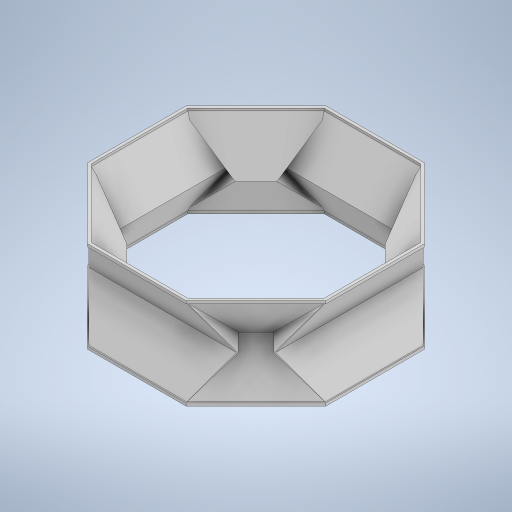
# Autodesk Inventor part: 팔각형 OV-PAM 층 한개
Saved by Autodesk Inventor 2024 (Build 280153000, 153)
## iProperties
Created: 2023-06-16
Part Number: 팔각형 OV-PAM 층 한개
Material: 일반
Document SubType Name: Modeling
Designer: jsw
Density: 1 g/cm^3
Appearance: 기본값
Author: jsw
Autodesk Inventor part; units mm, degrees
ref_plane "YZ Plane" through (0, 0, 0) normal (1, 0, 0) x (0, 1, 0)
ref_plane "XZ Plane" through (0, 0, 0) normal (0, 1, 0) x (-1, 0, 0)
ref_plane "XY Plane" through (0, 0, 0) normal (0, 0, 1) x (1, 0, 0)
sketch "스케치1" plane through (0, 0, 0) normal (0, 1, 0) x (-1, 0, 0)
  line L0 (-32.5919, 13.5) -> (-13.5, 32.5919)
  line L1 (-13.5, 32.5919) -> (13.5, 32.5919)
  line L2 (13.5, 32.5919) -> (32.5919, 13.5)
  line L3 (32.5919, 13.5) -> (32.5919, -13.5)
  line L4 (32.5919, -13.5) -> (13.5, -32.5919)
  line L5 (13.5, -32.5919) -> (-13.5, -32.5919)
  line L6 (-13.5, -32.5919) -> (-32.5919, -13.5)
  line L7 (-32.5919, -13.5) -> (-32.5919, 13.5)
  line L8 (-13.7071, 33.0919) -> (13.7071, 33.0919)
  line L9 (13.7071, 33.0919) -> (33.0919, 13.7071)
  line L10 (33.0919, 13.7071) -> (33.0919, -13.7071)
  line L11 (33.0919, -13.7071) -> (13.7071, -33.0919)
  line L12 (13.7071, -33.0919) -> (-13.7071, -33.0919)
  line L13 (-13.7071, -33.0919) -> (-33.0919, -13.7071)
  line L14 (-33.0919, -13.7071) -> (-33.0919, 13.7071)
  line L15 (-33.0919, 13.7071) -> (-13.7071, 33.0919)
  point P0 (0, 0)
  point P1 (0, 0)
  point P2 (0, 0)
  dimension "d0" = 27
  dimension "d2" = 0.5
  constraints: 32 end point, 2 coincident, 2 horizontal, 34 other
  measures "d0" distance of L0.end L1.end
  measures "d2" distance between parallel lines of L10 L3
extrude "돌출2" add sketch "스케치1" along normal blind 12 contours L0 L1 L2 L3 L4 L5 L6 L7 | L8 L9 L10 L11 L12 L13 L14 L15
ref_plane "작업 평면2" through (33.0919, 0, 13.7071) normal (-0.8660254, -0.5, 0) x (0, 0, -1)
sketch "스케치3" plane through (33.0919, 0, 13.7071) normal (1, 0, 0) x (0, 0, -1)
  line L0 (0, 0) -> (0, 12) projected
  line L1 (0, 12) -> (27.4142, 12) projected
  line L2 (0, 0) -> (27.4142, 0)
  line L3 (27.4142, 0) -> (27.4142, 12)
  line L4 (27.4142, 12) -> (0, 12)
  line L5 (0, 12) -> (0, 0)
  line L6 (0, 12) -> (-7.3047, 12)
  line L7 (-19.3848, 12) -> (0, 12) projected
  line L8 (0, 0) -> (-7.3047, 12)
  line L9 (27.4142, 12) -> (34.7189, 12)
  line L10 (34.7189, 12) -> (27.4142, 0)
  point P0 (13.7071, 0)
  dimension "d17" = 121.33
  dimension "d18" = 121.33
  constraints: 16 end point, 2 parallel, 2 point on line, 1 horizontal, 1 perpendicular
  measures "d17" angle of L8 L2
  measures "d18" angle of L2 L10
extrude "돌출4" cut sketch "스케치3" against normal up to surface surface through (33.0919, 0, 13.7071) normal (-0.8660254, -0.5, 0)
sketch "스케치4" plane through (13.7071, 0, 33.0919) normal (0.7071068, 0, 0.7071068) x (0.7071068, 0, -0.7071068)
  line L0 (0, 0) -> (0, 12) projected
  line L1 (27.4142, 0) -> (27.4142, 12) projected
  line L2 (0, 0) -> (27.4142, 0)
  line L3 (27.4142, 0) -> (27.4142, 12)
  line L4 (27.4142, 12) -> (0, 12)
  line L5 (0, 12) -> (0, 0)
  line L6 (27.4142, 0) -> (17.6163, 12) projected
  line L7 (27.4142, 0) -> (17.2071, 12)
  line L8 (27.4142, 0) -> (0, 0) projected
  line L9 (0, 0) -> (10.2071, 12)
  line L10 (27.4142, 12) -> (0, 12) projected
  point P0 (13.7071, 0)
  point P1 (13.7071, 12)
  dimension "d40" = 7
  dimension "d41" = 3.5
  constraints: 12 end point, 2 parallel, 2 point on line, 1 horizontal, 1 midpoint, 1 perpendicular
  measures "d40" distance of L9.end L7.end
  measures "d41" distance of L7.end point (13.707, 12)
ref_plane "작업 평면3" through (13.7071, 0, 33.0919) normal (0.6123724, 0.5, 0.6123724) x (0.7071068, 0, -0.7071068)
extrude "돌출5" cut sketch "스케치4" against normal up to surface contours L9 L4 L7 L2 surface through (13.7071, 0, 33.0919) normal (0.6123724, 0.5, 0.6123724)
pattern_circular "원형 패턴1" count 4 over 360 about axis through (0, -10, 0) along (0, 1, 0) of "돌출4"
pattern_circular "원형 패턴2" count 4 over 360 about axis through (0, -10, 0) along (0, 1, 0) of "돌출5"
mirror "미러5" about plane through (0, 12, 0) normal (0, 1, 0) of "돌출2", "돌출5", "원형 패턴2", "돌출4", "원형 패턴1"
ref_plane "작업 평면5" through (-13.7071, 12, -33.0919) normal (0, 1, 0) x (1, 0, 0)
sketch "스케치9" plane through (-13.7071, 24, -33.0919) normal (0, 1, 0) x (1, 0, 0)
  line L0 (46.799, -46.799) -> (46.799, -19.3848) projected
  line L1 (46.799, -19.3848) -> (27.4142, 0) projected
  line L2 (27.4142, 0) -> (0, 0) projected
  line L3 (0, 0) -> (-19.3848, -19.3848) projected
  line L4 (-19.3848, -19.3848) -> (-19.3848, -46.799) projected
  line L5 (-19.3848, -46.799) -> (0, -66.1838) projected
  line L6 (0, -66.1838) -> (27.4142, -66.1838) projected
  line L7 (27.4142, -66.1838) -> (46.799, -46.799) projected
  point P0 (13.7071, -33.0919)
extrude "돌출8" add sketch "스케치9" along normal blind 0.8
mirror "미러7" about plane through (-13.7071, 12, -33.0919) normal (0, 1, 0) of "돌출8"
shell "쉘5" thickness 0.5 removed faces 2 at (4.569, 24.8, 11.0306) at (4.569, -0.8, 11.0306)
sketch "스케치10" plane through (-13.7071, -0.8, 33.0919) normal (0, -1, 0) x (1, 0, 0)
  line L0 (-0.1243, 0.3) -> (27.5385, 0.3)
  line L1 (27.5385, 0.3) -> (47.099, -19.2605)
  line L2 (47.099, -19.2605) -> (47.099, -46.9233)
  line L3 (47.099, -46.9233) -> (27.5385, -66.4838)
  line L4 (27.5385, -66.4838) -> (-0.1243, -66.4838)
  line L5 (-0.1243, -66.4838) -> (-19.6848, -46.9233)
  line L6 (-19.6848, -46.9233) -> (-19.6848, -19.2605)
  line L7 (-19.6848, -19.2605) -> (-0.1243, 0.3)
  line L8 (46.799, -19.3848) -> (46.799, -46.799) projected
  line L9 (46.299, -19.5919) -> (46.299, -46.5919) projected
  line L10 (46.299, -46.5919) -> (27.2071, -65.6838) projected
  line L11 (27.2071, -65.6838) -> (0.2071, -65.6838) projected
  line L12 (0.2071, -65.6838) -> (-18.8848, -46.5919) projected
  line L13 (-18.8848, -46.5919) -> (-18.8848, -19.5919) projected
  line L14 (-18.8848, -19.5919) -> (0.2071, -0.5) projected
  line L15 (0.2071, -0.5) -> (27.2071, -0.5) projected
  line L16 (27.2071, -0.5) -> (46.299, -19.5919) projected
  line L17 (46.799, -46.799) -> (27.4142, -66.1838) projected
  line L18 (46.799, -19.3848) -> (46.799, -46.799) projected
  line L19 (27.4142, 0) -> (46.799, -19.3848) projected
  line L20 (0, 0) -> (27.4142, 0) projected
  line L21 (-19.3848, -19.3848) -> (0, 0) projected
  line L22 (-19.3848, -46.799) -> (-19.3848, -19.3848) projected
  line L23 (0, -66.1838) -> (-19.3848, -46.799) projected
  line L24 (27.4142, -66.1838) -> (0, -66.1838) projected
  point P0 (13.7071, -33.0919)
  point P1 (13.7071, -33.0919)
  dimension "d42" = 0.3
  constraints: 16 end point, 1 coincident, 1 horizontal, 17 other
  measures "d42" distance between parallel lines of L8 L2
extrude "돌출9" add sketch "스케치10" against normal blind 0.8 contours L0 L1 L2 L3 L4 L5 L6 L7
mirror "미러8" about plane through (-13.7071, 12, -33.0919) normal (0, 1, 0) of "돌출9"
equation "\"d41\" = 0.5 * d40"
